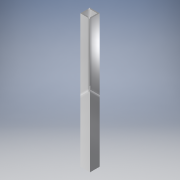
# Autodesk Inventor part: 15102898-16-P-0218
Saved by Autodesk Inventor 2017 (Build 210142000, 142)
## iProperties
Created: 2016-10-08
Part Number: 15102898-16-P-0218
Material: Aluminum 6061
Document SubType Name: Modeling
Designer: gus
Density: 2.7 g/cm^3
Appearance: Aluminum - Flat
Author: gus
Autodesk Inventor part; units mm, degrees
ref_plane "YZ Plane" through (0, 0, 0) normal (1, 0, 0) x (0, 1, 0)
ref_plane "XZ Plane" through (0, 0, 0) normal (0, 1, 0) x (-1, 0, 0)
ref_plane "XY Plane" through (0, 0, 0) normal (0, 0, 1) x (1, 0, 0)
sketch "Sketch1" plane through (0, 0, 0) normal (0, 1, 0) x (-1, 0, 0)
  line L0 (0, 0) -> (25.4, 0)
  line L1 (25.4, 0) -> (25.4, -25.4)
  line L2 (25.4, -25.4) -> (0, -25.4)
  line L3 (0, -25.4) -> (0, 0)
  line L4 (22.225, -22.225) -> (22.225, -3.175)
  line L5 (22.225, -3.175) -> (3.175, -3.175)
  line L6 (3.175, -3.175) -> (3.175, -22.225)
  line L7 (3.175, -22.225) -> (22.225, -22.225)
  dimension "d0" = 25.4
  dimension "d1" = 25.4
  dimension "d2" = 3.175
  constraints: 16 end point, 4 parallel, 2 perpendicular, 1 horizontal, 3 other
  measures "d0" distance of L1.end L2.end
  measures "d1" distance of L0.end L1.end
  measures "d2" distance between parallel lines of L1 L4
ref_plane "Work Plane1" through (-12.317, 252.2208, -280.054) normal (0, 1, 0) x (0, 0, 1)
ref_plane "Work Plane2" through (-12.317, 601.4708, -280.054) normal (0, -1, 0) x (1, 0, 0)
extrude "Extrusion1" add sketch "Sketch1" along normal up to surface (349.25 mm away) from surface at 252.2208
body "Solid1"
